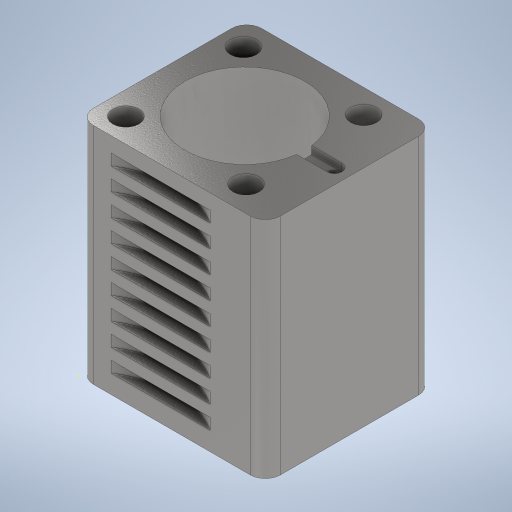
# Autodesk Inventor part: Piston_cilinder
Saved by Autodesk Inventor 2024 (Build 280153000, 153)
## iProperties
Created: 2023-11-02
Part Number: Piston_cilinder
Material: Ocel, pozinkovaná
Document SubType Name: Modeling
Designer: zak
Density: 7.85 g/cm^3
Appearance: Pozinkovaná
Author: zak
Autodesk Inventor part; units mm, degrees
ref_plane "YZ Plane" through (0, 0, 0) normal (1, 0, 0) x (0, 1, 0)
ref_plane "XZ Plane" through (0, 0, 0) normal (0, 1, 0) x (-1, 0, 0)
ref_plane "XY Plane" through (0, 0, 0) normal (0, 0, 1) x (1, 0, 0)
sketch "Náčrt3" plane through (0, 0, 0) normal (0, 1, 0) x (-1, 0, 0)
  line L0 (0, 0) -> (-50, 0)
  line L1 (-50, 0) -> (-50, -45)
  line L2 (-50, -45) -> (0, -45)
  line L3 (0, -45) -> (0, 0)
  line L4 (-22, 0) -> (-22, -45)
  line L5 (0, -22.5) -> (-50, -22.5)
  circle A0 centre (-22, -22.5) radius 16
  dimension "d0" = 50
  dimension "d1" = 45
  dimension "d2" = 22
  dimension "d3" = 32
  constraints: 12 end point, 3 midpoint, 3 point on line, 2 parallel, 2 perpendicular, 1 centre point, 1 horizontal
  measures "d0" distance of L2.end L1.end
  measures "d1" distance of L1.end L0.end
  measures "d2" distance between parallel lines of L3 L4
  measures "d3" diameter of A0
extrude "Vysunutí1" add sketch "Náčrt3" along normal blind 60 contours L3 L5 A0 L4 L0 | L4 A0 L5 L1 L0 | L3 L2 L4 A0 L5 | L5 A0 L4 L2 L1
fillet "Zaoblení1" radius 4 4 edges at (0, 30, -45) (0, 30, 0) (50, 30, -45) (50, 30, 0)
sketch "Náčrt9" plane through (0, 60, 0) normal (0, 1, 0) x (1, 0, 0)
  circle A0 centre (22, 22.5) radius 16 projected
  circle A1 centre (22, 22.5) radius 16 projected
  arc A2 (46, 0) -> (50, 4) centre (46, 4) ccw projected
  line L0 (50, 4) -> (50, 41) projected
  arc A3 (50, 41) -> (46, 45) centre (46, 41) ccw projected
  line L1 (46, 45) -> (4, 45) projected
  arc A4 (4, 45) -> (0, 41) centre (4, 41) ccw projected
  line L2 (0, 41) -> (0, 4) projected
  arc A5 (0, 4) -> (4, 0) centre (4, 4) ccw projected
  line L3 (4, 0) -> (46, 0) projected
  circle A6 centre (22, 22.5) radius 22.5
  line L4 (0, 0) -> (44, 45) construction
  line L5 (4, 0) -> (46, 0) construction
  line L6 (45.0114, 0) -> (0.7273, 43.2999) construction
  point P0 (6.2699, 6.4123)
  point P1 (5.9123, 38.2301)
  point P2 (37.7301, 38.5877)
  point P3 (38.0877, 6.7699)
  constraints: 6 point on line, 5 point on circle, 4 end point, 1 centre point, 1 coincident, 1 midpoint
hole "Díra1" at (6.2699, 60, -6.4123) at (5.9123, 60, -38.2301) at (37.7301, 60, -38.5877) at (38.0877, 60, -6.7699) direction (0, -1, 0) diameter 7 end through all
sketch "Náčrt10" plane through (0, 60, 0) normal (0, 1, 0) x (1, 0, 0)
  arc A0 (46, 20.5) -> (46, 24.5) centre (46, 22.5) ccw
  line L0 (0, 41) -> (0, 4) construction
  line L1 (0, 22.5) -> (50, 22.5) construction
  line L2 (50, 4) -> (50, 41) construction
  line L3 (22, 45) -> (22, 0) construction
  circle A1 centre (22, 22.5) radius 16 construction
  line L4 (46, 24.5) -> (37.8745, 24.5)
  line L5 (46, 20.5) -> (37.8745, 20.5)
  circle A2 centre (22, 22.5) radius 16 construction
  line L6 (46, 24.5) -> (46, 20.5)
  arc A3 (37.8745, 20.5) -> (37.8745, 24.5) centre (22, 22.5) ccw
  point P0 (0, 0)
  point P1 (38, 22.5)
  point P2 (6, 22.5)
  dimension "d58" = 4
  dimension "d59" = 24
  constraints: 10 end point, 9 point on circle, 3 point on line, 2 centre point, 2 midpoint, 1 coincident, 1 horizontal, 1 parallel, 1 perpendicular, 1 symmetric about line, 1 tangent, 1 vertical
  measures "d58" diameter of A0
  measures "d59" distance from line of A0.centre L3
extrude "Vysunutí6" cut sketch "Náčrt10" against normal blind 2
sketch "Náčrt12" plane through (0, 58, 0) normal (0, 1, 0) x (1, 0, 0)
  arc A0 (46, 20.5) -> (46, 24.5) centre (46, 22.5) ccw projected
  point P0 (0, 0)
  constraints: 1 coincident
hole "Díra2" at (46, 58, -22.5) direction (0, -1, 0) diameter 4 end through all
ref_plane "Pracovní rovina1" through (0, 56, 0) normal (0, 1, 0) x (1, 0, 0)
sketch "Náčrt13" plane through (0, 56, 0) normal (0, 1, 0) x (1, 0, 0)
  circle A0 centre (22, -20) radius 24
  circle A1 centre (22, 22.5) radius 16 construction
  line L0 (22, 38.5) -> (22, -52.7318) construction
  circle A2 centre (46, 22.5) radius 2 construction
  circle A3 centre (37.7301, 38.5877) radius 3.5 construction
  circle A4 centre (6.2699, 6.4123) radius 3.5 construction
  circle A5 centre (5.9123, 38.2301) radius 3.5 construction
  circle A6 centre (38.0877, 6.7699) radius 3.5 construction
  arc A7 (46, 0) -> (50, 4) centre (46, 4) ccw construction
  line L1 (4, 0) -> (46, 0) construction
  arc A8 (0, 4) -> (4, 0) centre (4, 4) ccw construction
  line L2 (0, 41) -> (0, 4) construction
  arc A9 (4, 45) -> (0, 41) centre (4, 41) ccw construction
  line L3 (46, 45) -> (4, 45) construction
  arc A10 (50, 41) -> (46, 45) centre (46, 41) ccw construction
  line L4 (50, 4) -> (50, 41) construction
  circle A11 centre (22, 22.5) radius 16 construction
  point P0 (0, 0)
  point P1 (22, 4)
  dimension "d70" = 48
  dimension "d71" = 20
  constraints: 3 point on line, 2 end point, 2 vertical alignment, 1 vertical, 3 other
  measures "d71" distance from line of L1 point (22, -20)
extrude "Vysunutí7" cut sketch "Náčrt13" against normal blind 3
pattern_circular "Kruhové pole1" count 4 over 360 about axis through (22, 0, -22.5) along (0, -1, 0) of "Vysunutí7" skipped copies 4
pattern_linear "Obdélníkové pole1" count 9 spacing 6 along (0, -1, 0) of "Vysunutí7", "Kruhové pole1"
sketch "Náčrt14" plane through (0, 0, 0) normal (0, -1, 0) x (1, 0, 0)
  point P0 (0, 0)
sketch "Náčrt15" plane through (0, 0, 0) normal (0, -1, 0) x (1, 0, 0)
  circle A0 centre (22, -22.5) radius 16 projected
  circle A1 centre (38.0877, -6.7699) radius 3.5 projected
  circle A2 centre (46, -22.5) radius 2 projected
  circle A3 centre (37.7301, -38.5877) radius 3.5 projected
  circle A4 centre (6.2699, -6.4123) radius 3.5 projected
  circle A5 centre (5.9123, -38.2301) radius 3.5 projected
  circle A6 centre (38.0877, -6.7699) radius 3.5 projected
  arc A7 (50, -4) -> (46, 0) centre (46, -4) ccw projected
  line L0 (4, 0) -> (46, 0) projected
  arc A8 (4, 0) -> (0, -4) centre (4, -4) ccw projected
  line L1 (0, -41) -> (0, -4) projected
  arc A9 (0, -41) -> (4, -45) centre (4, -41) ccw projected
  line L2 (46, -45) -> (4, -45) projected
  arc A10 (46, -45) -> (50, -41) centre (46, -41) ccw projected
  line L3 (50, -4) -> (50, -41) projected
  circle A11 centre (22, -22.5) radius 16 projected
  circle A12 centre (22, -22.5) radius 16
  circle A13 centre (22, -22.5) radius 18
  point P0 (0, 0)
  dimension "d80" = 36
  constraints: 2 centre point, 2 coincident, 1 concentric
  measures "d80" diameter of A13
extrude "Vysunutí8" add sketch "Náčrt15" along normal blind 2 contours A13
